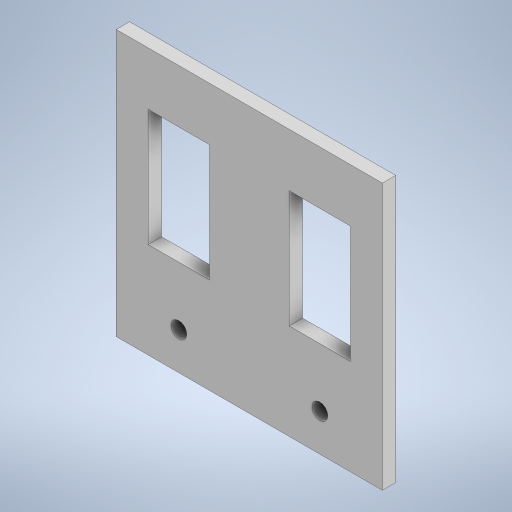
# Autodesk Inventor part: support_servo
Saved by Autodesk Inventor 2024 (Build 280153000, 153)
## iProperties
Created: 2023-10-09
Part Number: support_servo
Material: Générique
Document SubType Name: Modeling
Designer: apolline
Density: 1 g/cm^3
Appearance: Par défaut
Author: apolline
## iProperties of the stored document support_servo_Impression 3D.ipt
Created: 2023-10-09
Part Number: support_servo_Impression 3D
Material: Générique
Document SubType Name: Modeling
Designer: apolline
Density: 1 g/cm^3
Appearance: Par défaut
Author: apolline
Autodesk Inventor part; units mm, degrees
ref_plane "YZ Plane" through (0, 0, 0) normal (1, 0, 0) x (0, 1, 0)
ref_plane "XZ Plane" through (0, 0, 0) normal (0, 1, 0) x (-1, 0, 0)
ref_plane "XY Plane" through (0, 0, 0) normal (0, 0, 1) x (1, 0, 0)
sketch "Esquisse1" plane through (0, 0, 0) normal (0, 0, 1) x (1, 0, 0)
  line L0 (-50, -50) -> (50, -50)
  line L1 (50, -50) -> (50, 50)
  line L2 (50, 50) -> (-50, 50)
  line L3 (-50, 50) -> (-50, -50)
  line L4 (-50, -50) -> (50, 50) construction
  line L5 (50, -50) -> (-50, 50) construction
  line L6 (-38, 30) -> (-15, 30)
  line L7 (-15, 30) -> (-15, -14)
  line L8 (-15, -14) -> (-38, -14)
  line L9 (-38, -14) -> (-38, 30)
  line L10 (-38, 30) -> (-15, -14) construction
  line L11 (-15, 30) -> (-38, -14) construction
  line L12 (15, 30) -> (38, 30)
  line L13 (38, 30) -> (38, -14)
  line L14 (38, -14) -> (15, -14)
  line L15 (15, -14) -> (15, 30)
  line L16 (15, 30) -> (38, -14) construction
  line L17 (38, 30) -> (15, -14) construction
  circle A0 centre (-26.5, -36) radius 3
  circle A1 centre (26.5, -36) radius 3
  point P0 (0, 0)
  point P1 (-26.5, 8)
  point P2 (26.5, 8)
  point P3 (0, -50)
  dimension "d0" = 100
  dimension "d1" = 100
  dimension "d2" = 23
  dimension "d3" = 44
  dimension "d4" = 23
  dimension "d5" = 44
  dimension "d6" = 6
  dimension "d7" = 6
  dimension "d8" = 53
  dimension "d9" = 0
  dimension "d10" = 14
  dimension "d13" = 0
  dimension "d14" = 0
  dimension "d15" = 26.5
  dimension "d16" = 80
  dimension "d17" = 0
  constraints: 36 end point, 7 midpoint, 6 parallel, 3 horizontal, 3 perpendicular, 2 centre point
  measures "d0" distance of L1.end L2.end
  measures "d1" distance of L0.end L1.end
  measures "d2" distance of L6.start L6.end
  measures "d3" distance of L6.end L7.end
  measures "d4" distance of L12.start L12.end
  measures "d5" distance of L14.end L12.start
  measures "d6" diameter of A0
  measures "d7" diameter of A1
  measures "d8" distance of A1.centre A0.centre
  measures "d9" vertical distance of A1.centre A0.centre
  measures "d10" distance from line of L0 A0.centre
  measures "d13" horizontal distance of A0.centre point (-26.5, 8)
  measures "d14" horizontal distance of A1.centre point (26.5, 8)
  measures "d15" horizontal distance of point (0, -50) A0.centre
  measures "d16" distance between parallel lines of L0 L12
  measures "d17" distance between parallel lines of L6 L12
extrude "Extrusion1" add sketch "Esquisse1" along normal blind 5
